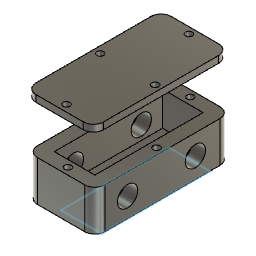
ECU_Casing-V1 v2 (Autodesk Fusion 360 design; units mm, degrees)
Autodesk Fusion 360 part; units mm, degrees
sketch "Sketch1" plane through (0, 0, 0) normal (0, 0, 1) x (1, 0, 0)
  line L0 (-15, 0) -> (-85, 0)
  line L1 (-100, 15) -> (-100, 185)
  line L2 (-85, 200) -> (-15, 200)
  line L3 (0, 185) -> (0, 15)
  arc A0 (-100, 15) -> (-85, 0) centre (-85, 15) ccw
  arc A1 (-85, 200) -> (-100, 185) centre (-85, 185) ccw
  arc A2 (0, 185) -> (-15, 200) centre (-15, 185) ccw
  arc A3 (-15, 0) -> (0, 15) centre (-15, 15) ccw
  circle A4 centre (-90, 100) radius 5
  circle A5 centre (-49.4897, 190.5376) radius 5
  circle A6 centre (-9.4422, 100.6136) radius 5
  circle A7 centre (-49.9525, 10.0759) radius 5
  dimension "d1" = 15
  dimension "d2" = 10
  dimension "d3" = 10
  dimension "d4" = 10
  dimension "d5" = 10
  constraint horizontal L0
  constraint vertical L1
  constraint horizontal L2
  constraint vertical L3
  constraint tangent L0 A0
  constraint tangent L1 A0
  constraint tangent L1 A1
  constraint tangent L2 A1
  constraint equal A0 A1
  constraint tangent L2 A2
  constraint tangent L3 A2
  constraint equal A0 A2
  constraint tangent L3 A3
  constraint tangent L0 A3
  constraint equal A0 A3
  measures "d1" radius of A0
  measures "d2" diameter of A4
  measures "d3" diameter of A5
  measures "d4" diameter of A6
  measures "d5" diameter of A7
extrude "Extrude1" add sketch "Sketch1" along normal blind 10 makes body 1
copy_body "CopyPasteBodies1" bodies 1 makes body 2
move_body "Move1" bodies 2 to x (1, 0, 0) y (0, 1, 0) z (0, 0, 1) at (-0.0948, -1.3287, 66.689)
move_body "Move2" bodies 2 to x (1, 0, 0) y (0, 1, 0) z (0, 0, 1) at (0, 0, -10)
move_body "Move3" bodies 2 to x (1, 0, 0) y (0, 1, 0) z (0, 0, 1) at (0, 0, 3.31)
move_body "Move4" bodies 2 to x (1, 0, 0) y (0, 1, 0) z (0, 0, 1) at (0.1548, 1.3079, 0)
extrude "Extrude2" add 1 faces at (-49.6137, 69.6039, 69.999) along direction (0, 0, 1) blind 50 on bodies 2 bodies 2
sketch "Sketch2" plane through (0, 0, 0) normal (0, 0, 1) x (1, 0, 0)
  line L0 (-10, 180) -> (-70, 180)
  line L1 (-70, 180) -> (-70, 20)
  line L2 (-70, 20) -> (-10, 20)
  line L3 (-10, 20) -> (-10, 180)
  constraint horizontal L0
  constraint perpendicular L0 L1
  constraint perpendicular L1 L2
  constraint perpendicular L0 L3
sketch "Sketch3" plane through (0, 0, 119.999) normal (0, 0, 1) x (-1, 0, 0)
  circle A0 centre (9.3822, -100.5928) radius 5
  circle A1 centre (89.94, -99.9793) radius 5
  circle A2 centre (49.4297, -190.5169) radius 5
  circle A3 centre (49.8925, -10.0552) radius 5
  arc A4 (99.94, -14.9793) -> (84.94, 0.0207) centre (84.94, -14.9793) ccw
  line L0 (84.94, 0.0207) -> (14.94, 0.0207)
  arc A5 (14.94, 0.0207) -> (-0.06, -14.9793) centre (14.94, -14.9793) ccw
  line L1 (-0.06, -14.9793) -> (-0.06, -184.9793)
  arc A6 (-0.06, -184.9793) -> (14.94, -199.9793) centre (14.94, -184.9793) ccw
  line L2 (14.94, -199.9793) -> (84.94, -199.9793)
  arc A7 (84.94, -199.9793) -> (99.94, -184.9793) centre (84.94, -184.9793) ccw
  line L3 (99.94, -184.9793) -> (99.94, -14.9793)
  line L4 (80, -180) -> (20, -180)
  line L5 (20, -180) -> (20, -20)
  line L6 (20, -20) -> (80, -20)
  line L7 (80, -20) -> (80, -180)
  constraint horizontal L4
  constraint vertical L5
  constraint horizontal L6
  constraint vertical L7
ref_plane "WorkPlane1" through (-50, 100, 59.999) normal (0, 0, 1) x (-1, 0, 0)
extrude "Extrude3" cut sketch "Sketch3" against normal blind 50 contours L4 L5 L6 L7 bodies 2
move_body "Move5" bodies 1 to x (1, 0, 0) y (0, 1, 0) z (0, 0, 1) at (-2.4957, 227.254, 145.7201)
hole "Hole1" at (-99.94, 52.8347, 88.9588) direction (1, 0, 0) diameter 30 depth 60 tip angle 118 bodies 2
hole "Hole2" at (-99.94, 148.5775, 90.1073) direction (1, 0, 0) diameter 30 depth 120 tip angle 118 bodies 2
delete_face "DeleteFace1" 1 faces at (-93.2933, 53.5823, 103.9402) on bodies 2
hole "Hole3" at (-99.94, 48.2751, 88.9298) direction (1, 0, 0) diameter 30 depth 120 tip angle 118 bodies 2
move_body "Move6" bodies 2 to x (1, 0, 0) y (0, 1, 0) z (0, 0, 1) at (0, 0, -50)
move_body "Move7" bodies 1 to x (1, 0, 0) y (0, 1, 0) z (0, 0, 1) at (-0.0379, -226.8101, -6.643)
named bodies: "ECU-Casing-Top", "ECU-Casing-Bottom"
